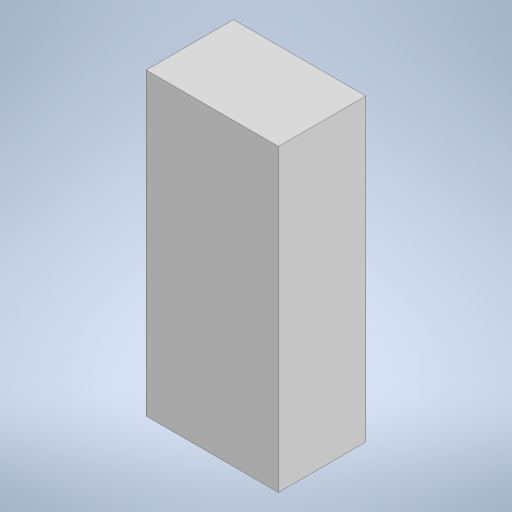
# Autodesk Inventor part: SwitchOnOff
Saved by Autodesk Inventor 2024 (Build 280153000, 153)
## iProperties
Created: 2023-11-16
Part Number: SwitchOnOff
Material: Générique
Document SubType Name: Modeling
Designer: digiacom
Density: 1 g/cm^3
Appearance: Par défaut
Author: digiacom
Autodesk Inventor part; units mm, degrees
ref_plane "YZ Plane" through (0, 0, 0) normal (1, 0, 0) x (0, 1, 0)
ref_plane "XZ Plane" through (0, 0, 0) normal (0, 1, 0) x (-1, 0, 0)
ref_plane "XY Plane" through (0, 0, 0) normal (0, 0, 1) x (1, 0, 0)
sketch "Esquisse1" plane through (0, 0, 0) normal (0, 1, 0) x (-1, 0, 0)
  line L0 (-3.1494, 4.7956) -> (0.3506, 4.7956)
  line L1 (0.3506, 4.7956) -> (0.3506, 3.0956)
  line L2 (0.3506, 3.0956) -> (-3.1494, 3.0956)
  line L3 (-3.1494, 3.0956) -> (-3.1494, 4.7956)
  line L4 (-4.0494, 5.6956) -> (1.2506, 5.6956)
  line L5 (1.2506, 5.6956) -> (1.2506, 2.1956)
  line L6 (1.2506, 2.1956) -> (-4.0494, 2.1956)
  line L7 (-4.0494, 2.1956) -> (-4.0494, 5.6956)
  point P0 (0, 0)
  dimension "d0" = 3.5
  dimension "d1" = 1.7
  dimension "d2" = 0.9
  dimension "d3" = 0.9
  dimension "d4" = 0.9
  dimension "d5" = 0.9
  constraints: 16 end point, 4 parallel, 2 horizontal, 2 perpendicular
  measures "d0" distance of L1.end L2.end
  measures "d1" distance of L0.end L1.end
  measures "d2" distance between parallel lines of L2 L6
  measures "d3" distance between parallel lines of L4 L0
  measures "d4" distance between parallel lines of L3 L7
  measures "d5" distance between parallel lines of L1 L5
extrude "Extrusion1" add sketch "Esquisse1" along normal blind 12
sketch "Esquisse2" plane through (0, 12, 0) normal (0, 1, 0) x (1, 0, 0)
  line L0 (3.1494, -4.7956) -> (-0.3506, -4.7956) projected
  line L1 (-0.3506, -4.7956) -> (3.1494, -4.7956)
  line L2 (3.1494, -4.7956) -> (3.1494, -3.0956)
  line L3 (3.1494, -3.0956) -> (-0.3506, -3.0956)
  line L4 (-0.3506, -3.0956) -> (-0.3506, -4.7956)
  point P0 (0, 0)
  constraints: 8 end point, 2 parallel, 1 horizontal, 1 perpendicular
extrude "Extrusion2" add sketch "Esquisse2" against normal blind 2
equation "\"d3\" = d2"
equation "\"d4\" = d2"
equation "\"d5\" = d2"
